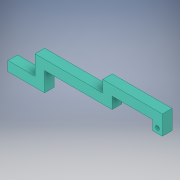
# Autodesk Inventor part: Arm
Saved by Autodesk Inventor 2018 (Build 220112000, 112)
## iProperties
Created: 2017-12-31
Part Number: Arm
Material: Generic
Document SubType Name: Modeling
Designer: suchanek
Density: 1 g/cm^3
Appearance: Default
Author: suchanek
Autodesk Inventor part; units mm, degrees
ref_plane "YZ Plane" through (0, 0, 0) normal (1, 0, 0) x (0, 1, 0)
ref_plane "XZ Plane" through (0, 0, 0) normal (0, 1, 0) x (-1, 0, 0)
ref_plane "XY Plane" through (0, 0, 0) normal (0, 0, 1) x (1, 0, 0)
sketch "Sketch1" plane through (0, 0, 0) normal (0, 0, 1) x (1, 0, 0)
  line L0 (0, 0) -> (14, 0)
  line L1 (14, 0) -> (14, 5)
  line L2 (14, 5) -> (0, 5)
  line L3 (0, 5) -> (0, 0)
  line L4 (14, 0) -> (19, 0)
  line L5 (19, 0) -> (19, 15)
  line L6 (19, 15) -> (14, 15)
  line L7 (14, 15) -> (14, 0)
  line L8 (19, 15) -> (49, 15)
  line L9 (49, 15) -> (49, 10)
  line L10 (49, 10) -> (19, 10)
  line L11 (19, 10) -> (19, 15)
  line L12 (49, 10) -> (54, 10)
  line L13 (54, 10) -> (54, 21)
  line L14 (54, 21) -> (49, 21)
  line L15 (49, 21) -> (49, 10)
  line L16 (54, 21) -> (80, 21)
  line L17 (80, 21) -> (80, 16)
  line L18 (80, 16) -> (54, 16)
  line L19 (54, 16) -> (54, 21)
  line L20 (80, 16) -> (75, 16)
  line L21 (75, 16) -> (75, 11)
  line L22 (75, 11) -> (80, 11)
  line L23 (80, 11) -> (80, 16)
  circle A0 centre (77.5, 13.5) radius 1
  dimension "d0" = 14
  dimension "d1" = 5
  dimension "d2" = 5
  dimension "d3" = 15
  dimension "d4" = 30
  dimension "d5" = 5
  dimension "d6" = 5
  dimension "d7" = 11
  dimension "d8" = 5
  dimension "d9" = 80
  dimension "d24" = 5
  dimension "d25" = 5
  dimension "d26" = 2
  dimension "d27" = 2.5
  dimension "d28" = 2.5
  constraints: 48 end point, 12 parallel, 6 horizontal, 6 perpendicular, 1 centre point
  measures "d0" distance of L2.end L1.end
  measures "d1" distance of L1.end L0.end
  measures "d2" distance of L6.end L5.end
  measures "d3" distance of L5.end L4.end
  measures "d4" distance of L9.end L10.end
  measures "d5" distance of L8.end L9.end
  measures "d6" distance of L14.end L13.end
  measures "d7" distance of L13.end L12.end
  measures "d8" distance of L16.end L17.end
  measures "d9" distance between parallel lines of L17 L3
  measures "d24" distance of L22.end L21.end
  measures "d25" distance of L21.end L20.end
  measures "d26" diameter of A0
  measures "d27" distance from line of L21 A0.centre
  measures "d28" distance from line of L22 A0.centre
extrude "Extrusion1" add sketch "Sketch1" along normal mid plane 5
body "Solid1"
